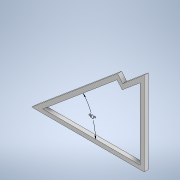
# Autodesk Inventor part: ballRampWithPocketForPowerCell
Saved by Autodesk Inventor 2020.2 (Build 242310000, 310)
## iProperties
Created: 2020-01-25
Part Number: ballRampWithPocketForPowerCell
Material: Generic
Document SubType Name: Modeling
Designer: robst
Density: 1 g/cm^3
Appearance: Default
Author: robst
Autodesk Inventor part; units mm, degrees
ref_plane "YZ Plane" through (0, 0, 0) normal (1, 0, 0) x (0, 1, 0)
ref_plane "XZ Plane" through (0, 0, 0) normal (0, 1, 0) x (-1, 0, 0)
ref_plane "XY Plane" through (0, 0, 0) normal (0, 0, 1) x (1, 0, 0)
sketch "Sketch1" plane through (0, 0, 0) normal (0, 0, 1) x (1, 0, 0)
  line L0 (0, 0) -> (544.8108, 457.1505)
  line L1 (0, 0) -> (749.0326, 0)
  line L2 (713.6671, 532.5231) -> (713.6671, 0)
  line L3 (713.6671, 532.5231) -> (577.4644, 418.2355)
  line L4 (577.4644, 418.2355) -> (544.8108, 457.1505)
  line L5 (69.7859, 25.4) -> (688.2671, 25.4)
  line L6 (688.2671, 25.4) -> (688.2671, 478.0527)
  line L7 (688.2671, 478.0527) -> (574.3337, 382.4512)
  line L8 (574.3337, 382.4512) -> (541.6801, 421.3662)
  line L9 (541.6801, 421.3662) -> (69.7859, 25.4)
  line L10 (688.2671, 511.21) -> (688.2671, 628.3123) construction
  line L11 (69.7859, 25.4) -> (39.5154, 0)
  line L12 (577.4644, 418.2355) -> (593.7912, 398.778) construction
  dimension "d10" = 40
  dimension "d12" = 532.5231
  dimension "d13" = 713.6671
  dimension "d14" = 177.8
  dimension "d15" = 711.2
  dimension "d16" = 50.8
  dimension "d17" = 25.4
  dimension "d18" = 25.4
  dimension "d19" = 25.4
  dimension "d20" = 25.4
  dimension "d21" = 25.4
  dimension "d32" = 618.4812
  dimension "d33" = 50
  dimension "d34" = 50
  dimension "d35" = 40
  dimension "d36" = 76.2
  dimension "d37" = 507.1231
  dimension "d38" = 674.1517
  dimension "d39" = 123.3295
  constraints: 26 end point, 6 perpendicular, 4 point on line, 3 parallel, 2 horizontal, 1 vertical
  measures "d10" angle of L0 L1
  measures "d12" distance of L2.start L2.end
  measures "d13" distance from line of L2 L0.start
  measures "d14" distance of L2.start L3.end
  measures "d15" distance of L0.start L0.end
  measures "d16" distance of L3.end L0.end
  measures "d17" distance between parallel lines of L5 L1
  measures "d18" distance between parallel lines of L6 L2
  measures "d19" distance between parallel lines of L0 L9
  measures "d20" distance between parallel lines of L8 L4
  measures "d21" distance between parallel lines of L3 L7
  measures "d32" distance of L5.end L5.start
  measures "d33" angle of L6 L7
  measures "d34" angle of L10 L3
  measures "d35" angle of L9 L5
  measures "d36" distance between parallel lines of L7 L0
  measures "d37" distance from line of L5 L2.start
  measures "d38" distance of L2.end L11.end
  measures "d39" distance of L12.end L6.end
extrude "Extrusion1" add sketch "Sketch1" along normal mid plane 25.4
ref_plane "planeForPowerCells" through (-48.9804, 58.3726, 12.7) normal (-0.6427876, 0.7660444, 0) x (0.7660444, 0.6427876, 0)
ref_plane "planeForShootingPowerCells" through (528.484, 476.6081, 12.7) normal (-0.6427876, 0.7660444, 0) x (0.7660444, 0.6427876, 0)
ref_plane "Work Plane3" through (612.9122, 514.2944, 12.7) normal (0.7660444, 0.6427876, 0) x (0, 0, -1)
body "Solid1"
